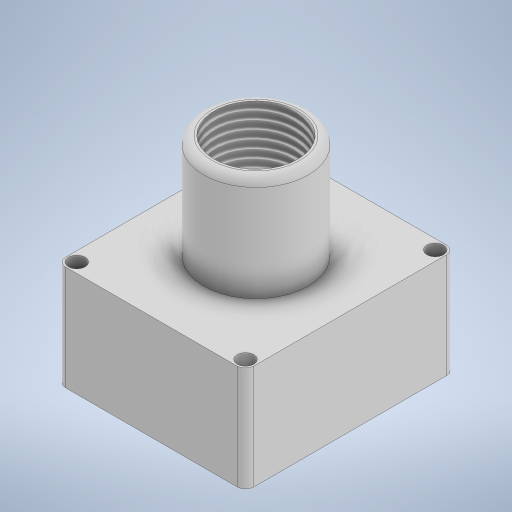
# Autodesk Inventor part: Tarea 01 Ayala Dinamica
Saved by Autodesk Inventor 2024 (Build 280153000, 153)
## iProperties
Created: 2024-02-19
Part Number: Tarea 01 Ayala Dinamica
Material: Genérico
Document SubType Name: Modeling
Designer: lejsa
Density: 1 g/cm^3
Appearance: Valor por defecto
Author: lejsa
Autodesk Inventor part; units mm, degrees
ref_plane "YZ Plane" through (0, 0, 0) normal (1, 0, 0) x (0, 1, 0)
ref_plane "XZ Plane" through (0, 0, 0) normal (0, 1, 0) x (-1, 0, 0)
ref_plane "XY Plane" through (0, 0, 0) normal (0, 0, 1) x (1, 0, 0)
sketch "Boceto1" plane through (0, 0, 0) normal (0, 1, 0) x (-1, 0, 0)
  line L0 (41, 50) -> (-41, 50)
  line L1 (-45, 46) -> (-45, -46)
  line L2 (-41, -50) -> (41, -50)
  line L3 (45, -46) -> (45, 46)
  line L4 (45, 50) -> (-45, -50) construction
  line L5 (-45, 50) -> (45, -50) construction
  arc A0 (45, 46) -> (41, 50) centre (41, 46) ccw
  arc A1 (41, -50) -> (45, -46) centre (41, -46) ccw
  arc A2 (-41, 50) -> (-45, 46) centre (-41, 46) ccw
  arc A3 (-45, -46) -> (-41, -50) centre (-41, -46) ccw
  line L6 (43.8284, -48.8284) -> (40.2929, -45.2929)
  line L7 (-43.8284, -48.8284) -> (-40.2929, -45.2929)
  line L8 (-43.8284, 48.8284) -> (-40.2929, 45.2929)
  circle A4 centre (-40.2929, 45.2929) radius 4
  line L9 (43.8284, 48.8284) -> (40.2929, 45.2929)
  circle A5 centre (40.2929, 45.2929) radius 4
  circle A6 centre (40.2929, -45.2929) radius 4
  circle A7 centre (-40.2929, -45.2929) radius 4
  point P0 (0, 0)
  dimension "d1" = 90
  dimension "d2" = 100
  dimension "d3" = 4
  dimension "d5" = 5
  dimension "d6" = 5
  dimension "d7" = 5
  dimension "d9" = 8
  dimension "d10" = 5
  dimension "d11" = 8
  dimension "d12" = 8
  dimension "d13" = 8
  constraints: 20 end point, 12 point on circle, 8 centre point, 8 point on line, 8 tangent, 4 coincident, 3 equal radius, 2 midpoint, 2 parallel, 1 horizontal, 1 perpendicular
  measures "d1" distance of L5.end L4.end
  measures "d2" distance of L4.end L5.start
  measures "d3" radius of A0
  measures "d5" distance of L6.start L6.end
  measures "d6" distance of L7.start L7.end
  measures "d7" distance of L8.start L8.end
  measures "d9" diameter of A4
  measures "d10" distance of L9.start L9.end
  measures "d11" diameter of A5
  measures "d12" diameter of A6
  measures "d13" diameter of A7
extrude "Extrusión1" add sketch "Boceto1" along normal blind 50
sketch "Boceto2" plane through (0, 50, 0) normal (0, 1, 0) x (1, 0, 0)
  circle A0 centre (0, 0) radius 25
  dimension "d16" = 50
  constraints: 1 centre point, 1 coincident
  measures "d16" diameter of A0
extrude "Extrusión2" add sketch "Boceto2" along normal blind 50
sketch "Boceto3" plane through (0, 100, 0) normal (0, 1, 0) x (1, 0, 0)
  circle A0 centre (0, 0) radius 20
  dimension "d19" = 40
  constraints: 1 centre point, 1 coincident
  measures "d19" diameter of A0
extrude "Extrusión3" cut sketch "Boceto3" against normal blind 30
thread "Rosca1" size "M50x4" class "6H" standard "ANSI Metric M Profile" full length
fillet "Empalme1" radius 4 1 edges at (-25, 100, 0)
